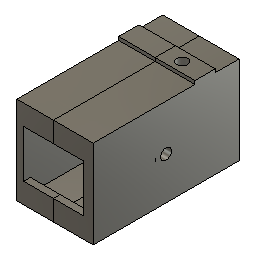
RJ45-Holder (Autodesk Fusion 360 design; units mm, degrees)
Autodesk Fusion 360 part; units mm, degrees
sketch "Sketch1" plane through (0, 0, 0) normal (1, 0, 0) x (0, 0, -1)
  line L0 (0, 0) -> (0, 26)
  line L1 (0, 26) -> (-43, 26)
  line L2 (-43, 26) -> (-43, 0)
  line L3 (-43, 0) -> (0, 0)
  line L4 (0, 2) -> (-43, 2)
  line L5 (0, 20) -> (-43, 20)
  line L6 (-18.5, 20) -> (-18.5, 6)
  line L7 (-24.5, 20) -> (-24.5, 6)
  line L8 (-2, 6) -> (-2, 2)
  line L9 (-41, 6) -> (-41, 2)
  line L10 (-7, 26) -> (-7, 27)
  line L11 (-7, 27) -> (-13, 27)
  line L12 (-13, 27) -> (-13, 26)
  line L13 (-20, 26) -> (-20, 20)
  circle A0 centre (-21.53, 12.5) radius 3
  circle A1 centre (-21.53, 12.5) radius 1.6
  line L14 (-24.5, 8.0245) -> (-18.5, 8.0245)
  line L15 (0, 6) -> (-18.5, 6)
  line L16 (-24.5, 6) -> (-43, 6)
  dimension "d1" = 26
  dimension "d2" = 43
  dimension "d3" = 2
  dimension "d4" = 6
  dimension "d5" = 4
  dimension "d6" = 18.5
  dimension "d7" = 18.5
  dimension "d8" = 2
  dimension "d9" = 2
  dimension "d10" = 6
  dimension "d11" = 7
  dimension "d12" = 20
  dimension "d13" = 6
  dimension "d14" = 3.2
  dimension "d32" = 1
  measures "d1" distance of L0.start L0.end
  measures "d2" distance of L0.start L2.end
  measures "d3" distance of L3 L4
  measures "d4" distance of L1 L5
  measures "d5" distance of L4 L15
  measures "d6" distance of L0 L6
  measures "d7" distance of L2 L7
  measures "d8" distance of L0 L8
  measures "d9" distance of L2 L9
  measures "d10" distance of L10.end L11.end
  measures "d11" distance of L0 L10
  measures "d12" distance of L0 L13
  measures "d13" diameter of A0
  measures "d14" diameter of A1
  measures "d32" distance of L1 L11
extrude "Extrude1" add sketch "Sketch1" against normal blind 2 contours L0 L2 L3 L4 | L0 L4 L8 L15 | L0 L5 L6 L15 | L4 L6 L7 L8 L9 L14 L15 L16 | L2 L4 L9 L16 | L0 L1 L5 L13 | L2 L5 L7 A0 L16 | L5 L6 L7 A0 L14 | L1 L2 L5 L13 | L1 L10 L11 L12 makes body 1
extrude "Extrude2" add sketch "Sketch1" along normal blind 8.75 contours L0 L2 L3 L4 | L0 L4 L8 L15 | L2 L4 L9 L16 | L0 L1 L5 L13 | L1 L2 L5 L13 | L1 L10 L11 L12 | L7 A0 | A1 picked at (-24.0433, 12.5) bodies 1
move_body "Move1" bodies 1 to x (1, 0, 0) y (0, 1, 0) z (0, 0, 1) at (-8.75, 0, 0)
extrude "Extrude3" add sketch "Sketch1" along normal blind 8.75 separate body contours L0 L2 L3 L4 | L0 L4 L8 L15 | L2 L4 L9 L16 | L0 L1 L5 L13 | L1 L2 L5 L13 | L1 L10 L11 L12 | L7 A0 | A1 picked at (-24.0433, 12.5) makes body 2 at (5.8333, 20, 14.3333) makes body 3 at (5.8333, 0, 28.6667) makes body 4 at (5.8333, 13.9383, 18.8973)
move_body "Move2" bodies 2 3 1 4 to x (1, 0, 0) y (0, 1, 0) z (0, 0, 1) at (-8.75, 0, 0)
extrude "Extrude4" add sketch "Sketch1" along normal blind 3 contours L0 L2 L3 L4 | L0 L4 L8 L15 | L0 L5 L6 L15 | L4 L6 L7 L8 L9 L14 L15 L16 | L2 L4 L9 L16 | L0 L1 L5 L13 | L2 L5 L7 A0 L16 | L5 L6 L7 A0 L14 | L1 L2 L5 L13 | L1 L10 L11 L12 | L7 A0 picked at (-24.0433, 12.5) bodies 4 2 3
move_body "Move3" bodies 4 1 to x (1, 0, 0) y (0, 1, 0) z (0, 0, 1) at (8.75, 0, 0)
extrude "Extrude5" add sketch "Sketch1" against normal blind 8.75 contours L5 L6 L7 A0 L14 bodies 1
extrude "Extrude6" cut sketch "Sketch1" against normal blind 10.75 contours A1 bodies 1
extrude "Extrude7" add sketch "Sketch1" along normal blind 8.75 contours L5 L6 L7 A0 L14 bodies 4
extrude "Extrude8" cut sketch "Sketch1" along normal blind 8.75 contours A1 bodies 4
sketch "Sketch2" plane through (0, 27, 0) normal (0, 1, 0) x (-1, 0, 0)
  line L0 (0, 7) -> (0, 13)
  line L1 (0, 13) -> (-11.75, 13)
  line L2 (-11.75, 13) -> (-11.75, 7)
  line L3 (-11.75, 7) -> (0, 7)
  circle A0 centre (-5, 10) radius 1.6
  circle A1 centre (-5, 10) radius 3
  dimension "d33" = 3.2
  dimension "d34" = 6
  measures "d33" diameter of A0
  measures "d34" diameter of A1
extrude "Extrude9" cut sketch "Sketch2" against normal up to surface (27 mm away) contours A0 bodies 4
sketch "Sketch3" plane through (0, 20, 0) normal (0, -1, 0) x (1, 0, 0)
  line L0 (0, 18.5) -> (0, 0)
  line L1 (0, 0) -> (8.75, 0)
  circle A0 centre (5, 10) radius 2.875
  line L2 (8.75, 0) -> (8.75, 18.5)
  circle A1 centre (5, 10) radius 1.6
  line L3 (8.75, 18.5) -> (0, 18.5)
  dimension "d37" = 5.75
  measures "d37" diameter of A0
extrude "Extrude10" cut sketch "Sketch3" against normal blind 3 contours A0 | A1 bodies 4
equation "d17 = ( 17.5 / 2 ) * 1 mm"
equation "d19 = ( 17.5 / 2 ) * 1 mm"
named bodies: "Right", "Left"
